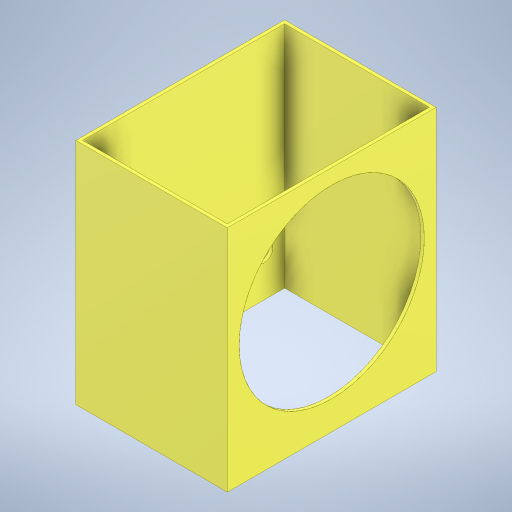
# Autodesk Inventor part: 7-32
Saved by Autodesk Inventor 2024 (Build 280153000, 153)
## iProperties
Created: 2024-11-09
Part Number: 7-32
Material: Latón, amarillo claro
Document SubType Name: Modeling
Designer: araya
Density: 8.47 g/cm^3
Appearance: Suave - Amarillo
Author: araya
Autodesk Inventor part; units mm, degrees
ref_plane "YZ Plane" through (0, 0, 0) normal (1, 0, 0) x (0, 1, 0)
ref_plane "XZ Plane" through (0, 0, 0) normal (0, 1, 0) x (-1, 0, 0)
ref_plane "XY Plane" through (0, 0, 0) normal (0, 0, 1) x (1, 0, 0)
sketch "Boceto1" plane through (0, 0, 0) normal (0, 1, 0) x (-1, 0, 0)
  line L0 (0, 0) -> (45, 0)
  line L1 (45, 0) -> (45, 62)
  line L2 (45, 62) -> (0, 62)
  line L3 (0, 62) -> (0, 0)
  line L4 (44, 61) -> (1, 61)
  line L5 (1, 61) -> (1, 1)
  line L6 (1, 1) -> (44, 1)
  line L7 (44, 1) -> (44, 61)
  point P0 (22.5, 62)
  dimension "d0" = 1
  dimension "d1" = 1
  dimension "d2" = 1
  dimension "d3" = 1
  dimension "d4" = 43
  dimension "d5" = 60
  constraints: 16 end point, 4 parallel, 2 horizontal, 2 perpendicular, 1 midpoint
  measures "d0" distance between parallel lines of L7 L1
  measures "d1" distance between parallel lines of L3 L5
  measures "d2" distance between parallel lines of L0 L6
  measures "d3" distance from line of point (22.5, 62) L4
  measures "d4" distance of L4.start L4.end
  measures "d5" distance of L4.end L5.end
extrude "Extrusión1" add sketch "Boceto1" along normal blind 68
sketch "Boceto2" plane through (0, 0, 62) normal (1, 0, 0) x (0, 0, -1)
  line L0 (0, 0) -> (62, 0) projected
  line L1 (62, 0) -> (62, 68) projected
  line L2 (0, 68) -> (62, 68) projected
  line L3 (0, 0) -> (0, 68) projected
  circle A0 centre (31, 36) radius 27.5
  point P0 (31, 68)
  dimension "d8" = 36
  dimension "d9" = 55
  constraints: 1 centre point, 1 midpoint, 1 vertical alignment
  measures "d8" vertical distance of L0.start A0.centre
  measures "d9" diameter of A0
hole "Agujero1" at (0, 36, 31) direction (-1, 0, 0) diameter 55 depth 1
sketch "Boceto3" plane through (-45, 0, 0) normal (-1, 0, 0) x (0, 0, 1)
  line L0 (0, 0) -> (62, 0) projected
  line L1 (62, 0) -> (62, 68) projected
  line L2 (0, 68) -> (62, 68) projected
  line L3 (0, 0) -> (0, 68) projected
  circle A0 centre (31, 12) radius 2.5
  circle A1 centre (7, 12) radius 2.5
  circle A2 centre (55, 12) radius 2.5
  circle A3 centre (15, 12) radius 2.5
  circle A4 centre (23, 12) radius 2.5
  circle A5 centre (39, 12) radius 2.5
  circle A6 centre (47, 12) radius 2.5
  point P0 (0, 0)
  point P1 (31, 68)
  dimension "d17" = 5
  dimension "d18" = 12
  dimension "d19" = 5
  dimension "d20" = 5
  dimension "d21" = 24
  dimension "d22" = 48
  dimension "d24" = 3
  dimension "d25" = 3
  dimension "d26" = 3
  dimension "d27" = 3
  dimension "d28" = 3
  constraints: 7 centre point, 6 horizontal alignment, 4 equal radius, 1 midpoint, 1 vertical alignment
  measures "d17" diameter of A0
  measures "d18" vertical distance of L0.end A0.centre
  measures "d19" diameter of A1
  measures "d20" diameter of A2
  measures "d21" distance of A1.centre A0.centre
  measures "d22" distance of A2.centre A1.centre
hole "Agujero2" at (-45, 12, 7) at (-45, 12, 15) at (-45, 12, 23) at (-45, 12, 31) at (-45, 12, 39) at (-45, 12, 47) at (-45, 12, 55) direction (1, 0, 0) diameter 5 depth 1
